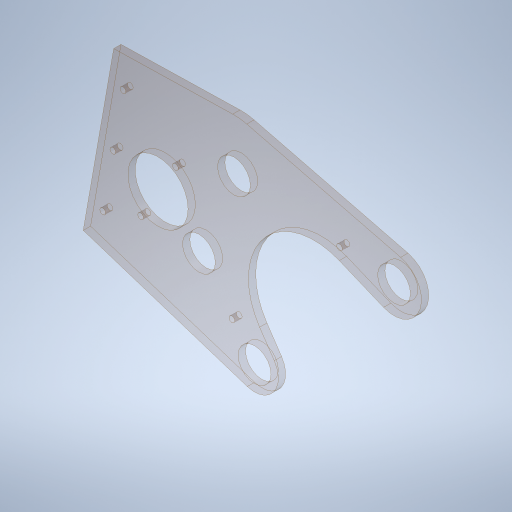
# Autodesk Inventor part: GP7-002
Saved by Autodesk Inventor 2023.4 (Build 274418000, 418)
## iProperties
Created: 2025-02-24
Part Number: GP7-002
Material: Polycarbonate, Smoke
Document SubType Name: Modeling
Designer: dlangdon
Density: 1.2 g/cm^3
Appearance: Polycarbonate - Smoked
Author: dlangdon
Autodesk Inventor part; units mm, degrees
ref_plane "YZ Plane" through (0, 0, 0) normal (1, 0, 0) x (0, 1, 0)
ref_plane "XZ Plane" through (0, 0, 0) normal (0, 1, 0) x (-1, 0, 0)
ref_plane "XY Plane" through (0, 0, 0) normal (0, 0, 1) x (1, 0, 0)
sketch "Sketch1" plane through (0, 0, 0) normal (0, 0, 1) x (1, 0, 0)
  circle A0 centre (65.1069, 65.1069) radius 38.1 construction
  circle A1 centre (-56.1266, -56.1266) radius 25.4 construction
  circle A2 centre (0, 0) radius 53.975 construction
  line L0 (-38.1661, -38.1661) -> (38.1661, 38.1661) construction
  line L1 (65.1069, 65.1069) -> (-56.1266, -56.1266) construction
  line L2 (-4.3707, 6.2419) -> (-4.3707, 53.7978) construction
  line L3 (-213.7801, -81.5266) -> (651.612, -81.5266) construction
  circle A3 centre (160.9403, -24.3766) radius 57.15 construction
  circle A4 centre (65.1069, 65.1069) radius 14.2875
  circle A5 centre (-56.1266, -56.1266) radius 14.2875
  circle A6 centre (-4.3707, 6.2419) radius 57.15 construction
  circle A7 centre (-56.1266, -56.1266) radius 20.6375 construction
  circle A8 centre (65.1069, 65.1069) radius 23.8125 construction
  circle A9 centre (-74.0632, 76.9679) radius 14.2875
  line L4 (-74.0632, 76.9679) -> (65.1069, 65.1069) construction
  circle A10 centre (65.1069, 65.1069) radius 14.3256 construction
  circle A11 centre (-56.1266, -56.1266) radius 14.3256 construction
  circle A12 centre (-104.5284, 3.6446) radius 14.2875
  line L5 (-56.1266, -56.1266) -> (-104.5284, 3.6446) construction
  circle A13 centre (-104.5284, 3.6446) radius 39.7002 construction
  circle A14 centre (-74.0632, 76.9679) radius 39.7002 construction
  line L6 (17.4877, 59.0466) -> (55.9992, 43.1049)
  line L7 (-39.0193, -44.5834) -> (-51.7448, -25.7239)
  arc A15 (17.4877, 59.0466) -> (-51.7448, -25.7239) centre (-4.3707, 6.2419) ccw
  line L8 (-178.6215, 120.6011) -> (-153.6074, 116.1905) construction
  line L9 (-153.6074, 116.1905) -> (-180.0714, -33.8943) construction
  line L10 (-180.0714, -33.8943) -> (-205.0855, -29.4836) construction
  line L11 (-205.0855, -29.4836) -> (-178.6215, 120.6011) construction
  line L12 (-209.5607, -54.8639) -> (48.3201, -100.3352) construction
  line L13 (-174.1463, 145.9814) -> (151.5491, 88.5525) construction
  line L14 (-174.1463, 145.9814) -> (-209.5607, -54.8639) construction
  circle A16 centre (-140.1331, 32.2196) radius 25.4 construction
  circle A17 centre (-140.1331, 32.2196) radius 5.9531 construction
  line L15 (-79.5442, -27.2082) -> (-72.1113, -36.3871) construction
  circle A18 centre (17.6539, 69.1511) radius 9.525 construction
  line L16 (-166.1144, 118.3958) -> (-192.5784, -31.6889) construction
  line L17 (-170.5251, 93.3817) -> (-188.1678, -6.6748) construction
  circle A19 centre (-140.1331, 32.2196) radius 17.4625 construction
  circle A20 centre (-140.1331, 32.2196) radius 9.525 construction
  circle A21 centre (-74.0632, 76.9679) radius 46.0502 construction
  line L18 (-178.6215, 120.6011) -> (-75.1329, 123.0056)
  line L19 (-62.8974, 121.6439) -> (70.8807, 88.2088)
  line L20 (-62.4968, -75.7563) -> (-205.0855, -29.4836)
  line L21 (-178.6215, 120.6011) -> (-205.0855, -29.4836)
  arc A22 (-62.8974, 121.6439) -> (-75.1329, 123.0056) centre (-74.0632, 76.9679) ccw
  arc A23 (55.9992, 43.1049) -> (70.8807, 88.2088) centre (65.1069, 65.1069) ccw
  arc A24 (-62.4968, -75.7563) -> (-39.0193, -44.5834) centre (-56.1266, -56.1266) ccw
  line L22 (-140.1331, 32.2196) -> (-131.4018, 47.3426) construction
  line L23 (-125.0518, 58.3411) -> (-155.2143, 6.0981) construction
  circle A25 centre (-155.2143, 6.0981) radius 4.7625 construction
  line L24 (-4.3707, 6.2419) -> (0, 0) construction
  circle A26 centre (-74.0632, 76.9679) radius 40.4812 construction
  circle A27 centre (-104.5284, 3.6446) radius 40.4812 construction
  circle A28 centre (-140.1331, 32.2196) radius 26.1938
  point P0 (-191.8535, 45.5588)
  point P1 (-75.8278, -31.7977)
  point P2 (-179.3464, 43.3534)
  point P3 (-179.3464, 43.3534)
  point P4 (-148.8643, 47.3426)
  point P5 (-157.5956, 32.2196)
  point P6 (-148.8643, 17.0967)
  point P7 (-131.4018, 17.0967)
  point P8 (-122.6706, 32.2196)
  point P9 (-63.3695, 121.1474)
  dimension "d7" = 50.8
  dimension "d18" = 79.4004
  dimension "d34" = 34.925
  dimension "d3" = 45
  dimension "d4" = 0
  dimension "d8" = 107.95
  dimension "d9" = 28.575
  dimension "d10" = 76.2
  dimension "d11" = 114.3
  dimension "d12" = 114.3
  dimension "d13" = 6.35
  dimension "d14" = 9.525
  dimension "d15" = 139.6746
  dimension "d16" = 28.6512
  dimension "d17" = 76.9112
  dimension "d19" = 79.4004
  dimension "d22" = 25.4
  dimension "d23" = 152.4
  dimension "d26" = 203.9436
  dimension "d27" = 50.8
  dimension "d28" = 11.9062
  dimension "d29" = 51
  dimension "d30" = 171.45
  dimension "d31" = 10
  dimension "d32" = 19.05
  dimension "d33" = 101.6
  dimension "d35" = 19.05
  dimension "d36" = 6.35
  dimension "d37" = 28.575
  dimension "d40" = 360
  dimension "d43" = 20
  dimension "d44" = 9.525
  dimension "d54" = 7.62
  dimension "d55" = 80
  dimension "d57" = 80.9625
  dimension "d59" = 0.7937
  constraints: 50 end point, 26 centre point, 24 coincident, 19 point on circle, 13 tangent, 9 midpoint, 6 equal radius, 4 collinear, 4 parallel, 4 point on line, 2 horizontal, 1 concentric, 1 perpendicular, 1 vertical, 20 other
  measures "d3" angle of L2 L0
  measures "d4" distance between parallel lines of L0 L1
  measures "d8" diameter of A2
  measures "d9" diameter of A4
  measures "d10" diameter of A0
  measures "d11" diameter of A3
  measures "d12" diameter of A6
  measures "d13" radial gap between concentric circles of A5 A7
  measures "d14" radial gap between concentric circles of A4 A8
  measures "d15" distance of L4.start L4.end
  measures "d16" diameter of A10
  measures "d17" distance of L5.start L5.end
  measures "d19" diameter of A14
  measures "d22" distance of L9.end L10.end
  measures "d23" distance of L10.end L8.start
  measures "d26" distance of L13.start L12.start
  measures "d27" diameter of A16
  measures "d28" diameter of A17
  measures "d29" angle of L3 L5
  measures "d30" distance from line of point (0, 0) L9
  measures "d31" angle of L3 L12
  measures "d32" diameter of A18
  measures "d33" distance of L17.start L17.end
  measures "d35" diameter of A20
  measures "d36" radial gap between concentric circles of A14 A21
  measures "d37" vertical distance of L5.end A16.centre
  measures "d43" angle of L9 L22
  measures "d44" diameter of A25
  measures "d54" distance of L2.start L24.end
  measures "d55" angle of L0 L24
  measures "d57" diameter of A26
  measures "d59" radial gap between concentric circles of A28 A16
extrude "Extrusion1" add sketch "Sketch1" along normal blind 6.35
hole "Hole1" at (-75.8278, -31.7977, 0) at (17.6539, 69.1511, 0) at (-170.5251, 93.3817, 0) at (-179.3464, 43.3534, 0) at (-188.1678, -6.6748, 0) at (-131.4018, 47.3426, 0) at (-148.8643, 47.3426, 0) at (-157.5956, 32.2196, 0) at (-148.8643, 17.0967, 0) at (-131.4018, 17.0967, 0) at (-122.6706, 32.2196, 0) at (-125.0518, 58.3411, 0) at (-155.2143, 6.0981, 0) direction (0, 0, 1) diameter 5.1054 end through all clearance for "Flat Head Machine Screw (82)" size "#10" standard "Ansi Unified Screw Threads"
body "Solid1"
